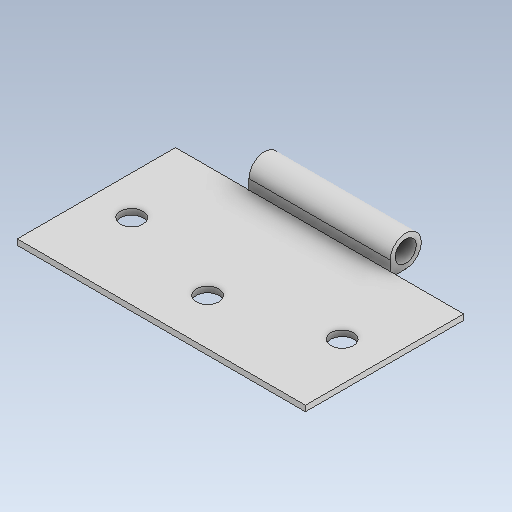
# Autodesk Inventor part: Ala 2 Bisagra tipo Libro Grande
Saved by Autodesk Inventor 2020 (Build 240168000, 168)
## iProperties
Created: 2020-07-02
Part Number: Ala 2 Bisagra tipo Libro Grande
Material: Genérico
Document SubType Name: Modeling
Designer: Pipi
Density: 1 g/cm^3
Appearance: Valor por defecto
Author: Pipi
Autodesk Inventor part; units mm, degrees
ref_plane "YZ Plane" through (0, 0, 0) normal (1, 0, 0) x (0, 1, 0)
ref_plane "XZ Plane" through (0, 0, 0) normal (0, 1, 0) x (-1, 0, 0)
ref_plane "XY Plane" through (0, 0, 0) normal (0, 0, 1) x (1, 0, 0)
sketch "Boceto1" plane through (0, 0, 0) normal (0, 1, 0) x (-1, 0, 0)
  line L0 (11.708, 26.8389) -> (11.708, -1.1611)
  line L1 (11.708, -1.1611) -> (-39.292, -1.1611)
  line L2 (-39.292, -1.1611) -> (-39.292, 26.8389)
  line L3 (-39.292, 26.8389) -> (11.708, 26.8389)
  circle A0 centre (4.833, 13.4639) radius 2
  circle A1 centre (-32.417, 13.4639) radius 2
  circle A2 centre (-13.792, 18.6686) radius 2
  point P0 (0, 0)
  point P1 (0, 0)
  dimension "d0" = 28
  dimension "d1" = 51
  dimension "d2" = 4
  dimension "d3" = 4
  dimension "d4" = 4
  dimension "d5" = 25.5
  dimension "d6" = 6.875
  dimension "d7" = 13.375
  dimension "d8" = 6.875
  dimension "d9" = 13.375
  constraints: 8 end point, 3 centre point, 3 perpendicular, 1 vertical
  measures "d0" distance of L0.start L0.end
  measures "d1" distance of L0.end L1.end
  measures "d2" diameter of A0
  measures "d3" diameter of A1
  measures "d4" diameter of A2
  measures "d5" distance from line of L0 A2.centre
  measures "d6" distance from line of L2 A1.centre
  measures "d7" distance from line of L3 A1.centre
  measures "d8" distance from line of L0 A0.centre
  measures "d9" distance from line of L3 A0.centre
extrude "Extrusión1" add sketch "Boceto1" along normal blind 1
sketch "Boceto2" plane through (39.292, 0, 26.8389) normal (1, 0, 0) x (0, 0, -1)
  arc A0 (30.75, 0) -> (28, 2.75) centre (30.75, 2.75) ccw
  circle A1 centre (30.75, 2.75) radius 1.875
  line L0 (0, 0) -> (28, 0) projected
  line L1 (28, 0) -> (28, 1) projected
  line L2 (28, 0) -> (30.75, 0)
  line L3 (28, 0) -> (28, 2.75)
  point P0 (26.8389, 0)
  dimension "d12" = 5.5
  dimension "d13" = 3.75
  constraints: 4 end point, 3 tangent, 2 centre point, 2 point on circle, 1 coincident, 1 perpendicular
  measures "d12" diameter of A0
  measures "d13" diameter of A1
extrude "Extrusión2" add sketch "Boceto2" against normal blind 38
sketch "Boceto3" plane through (39.292, 0, 26.8389) normal (1, 0, 0) x (0, 0, -1)
  circle A0 centre (30.75, 2.75) radius 1.875 projected
  arc A1 (30.75, 0) -> (28, 2.75) centre (30.75, 2.75) ccw
  arc A2 (30.75, 0) -> (28, 2.75) centre (30.75, 2.75) ccw projected
  line L0 (28, 2.75) -> (28, 0)
  line L1 (28, 0) -> (30.75, 0)
  point P0 (26.8389, 0)
  constraints: 4 end point, 3 tangent, 2 point on circle, 1 centre point, 1 coincident, 1 perpendicular, 1 vertical
extrude "Extrusión3" cut sketch "Boceto3" against normal blind 13
